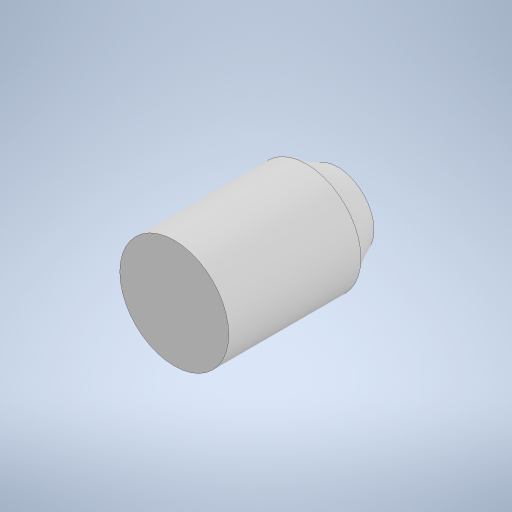
# Autodesk Inventor part: Shaft Adapter
Saved by Autodesk Inventor 2024 (Build 280153000, 153)
## iProperties
Created: 2024-01-26
Part Number: Shaft Adapter
Material: Generic
Document SubType Name: Modeling
Designer: aidan
Density: 1 g/cm^3
Appearance: Default
Author: aidan
Autodesk Inventor part; units mm, degrees
ref_plane "YZ Plane" through (0, 0, 0) normal (1, 0, 0) x (0, 1, 0)
ref_plane "XZ Plane" through (0, 0, 0) normal (0, 1, 0) x (-1, 0, 0)
ref_plane "XY Plane" through (0, 0, 0) normal (0, 0, 1) x (1, 0, 0)
sketch "Sketch1" plane through (0, 0, 0) normal (0, 0, 1) x (1, 0, 0)
  circle A0 centre (0, 0) radius 2.5
  line L0 (-1.3162, -2.1255) -> (1.3162, -2.1255)
  circle A1 centre (0, 0) radius 3.175
  dimension "d0" = 5
  dimension "d1" = 6.35
  constraints: 2 centre point, 2 coincident, 2 end point, 2 point on circle, 1 horizontal
  measures "d0" diameter of A0
  measures "d1" diameter of A1
extrude "Extrusion1" add sketch "Sketch1" along normal blind 6.35 contours L0 A0 | A1 picked at (-0.2721, -2.2046)
sketch "Sketch2" plane through (0, 0, 6.35) normal (0, 0, 1) x (1, 0, 0)
  circle A0 centre (0, 0) radius 9.525
  circle A1 centre (0, 0) radius 10.8857
  dimension "d4" = 19.05
  dimension "d5" = 21.7714
  constraints: 2 centre point, 2 coincident
  measures "d4" diameter of A0
  measures "d5" diameter of A1
extrude "Extrusion2" add sketch "Sketch2" along normal blind 6.35
sketch "Sketch4" plane through (0, 0, 12.7) normal (0, 0, 1) x (1, 0, 0)
  circle A0 centre (0, 0) radius 10.8857 projected
  circle A1 centre (0, 0) radius 9.525 projected
extrude "Extrusion4" add sketch "Sketch4" along normal blind 1.5875 contours A1
sketch "Sketch5" plane through (0, 0, 12.7) normal (0, 0, 1) x (1, 0, 0)
  circle A0 centre (0, 0) radius 10.8857 projected
  circle A1 centre (0, 0) radius 9.525 projected
extrude "Extrusion5" cut sketch "Sketch5" against normal blind 9.525
sketch "Sketch6" plane through (0, 0, 12.7) normal (0, 0, -1) x (-1, 0, 0)
  circle A0 centre (0, 0) radius 9.525 projected
extrude "Extrusion6" add sketch "Sketch6" along normal blind 6.477
fillet "Fillet2" radius 11.1125 1 edges at (-3.175, 0, 6.223)
sketch "Sketch7" plane through (0, 0, 14.2875) normal (0, 0, 1) x (1, 0, 0)
  circle A0 centre (0, 0) radius 9.525 projected
  circle A1 centre (0, 0) radius 4.7625
  dimension "d18" = 9.525
  constraints: 1 centre point, 1 coincident
  measures "d18" diameter of A1
extrude "Extrusion7" cut sketch "Sketch7" against normal blind 15.748
body "Solid1"
